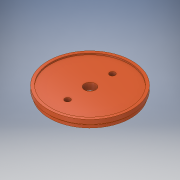
# Autodesk Inventor part: upper_thermal_barrier
Saved by Autodesk Inventor 2017 SP1 (Build 210196100, 196)
## iProperties
Created: 2016-10-21
Part Number: upper_thermal_barrier
Material: Phenolic Resin
Document SubType Name: Modeling
Designer: cflannery
Density: 1.38 g/cm^3
Appearance: Smooth - Light Orange
Author: cflannery
Autodesk Inventor part; units mm, degrees
ref_plane "YZ Plane" through (0, 0, 0) normal (1, 0, 0) x (0, 1, 0)
ref_plane "XZ Plane" through (0, 0, 0) normal (0, 1, 0) x (-1, 0, 0)
ref_plane "XY Plane" through (0, 0, 0) normal (0, 0, 1) x (1, 0, 0)
sketch "Sketch1" plane through (0, 0, 0) normal (0, 1, 0) x (-1, 0, 0)
  circle A0 centre (0, 0) radius 92.075
  dimension "d0" = 184.15
  constraints: 1 centre point, 1 coincident
  measures "d0" diameter of A0
extrude "Extrusion1" add sketch "Sketch1" along normal blind 6.35
sketch "Sketch2" plane through (0, 6.35, 0) normal (0, 1, 0) x (1, 0, 0)
  circle A0 centre (0, 0) radius 88.9
  dimension "d3" = 177.8
  constraints: 1 centre point, 1 coincident
  measures "d3" diameter of A0
extrude "Extrusion2" add sketch "Sketch2" along normal blind 3.175
sketch "Sketch3" plane through (0, 9.525, 0) normal (0, 1, 0) x (1, 0, 0)
  circle A0 centre (0, 0) radius 95.25
  dimension "d6" = 190.5
  constraints: 1 centre point, 1 coincident
  measures "d6" diameter of A0
extrude "Extrusion3" add sketch "Sketch3" along normal blind 6.35
sketch "Sketch8" plane through (0, 15.875, 0) normal (0, 1, 0) x (1, 0, 0)
  circle A0 centre (0, 0) radius 95.25
  circle A1 centre (0, 0) radius 88.9
  dimension "d33" = 177.8
  dimension "d34" = 190.5
  constraints: 2 centre point, 2 coincident
  measures "d33" diameter of A1
  measures "d34" diameter of A0
extrude "Extrusion9" add sketch "Sketch8" along normal blind 3.175
sketch "Sketch9" plane through (0, 15.875, 0) normal (0, 1, 0) x (1, 0, 0)
  circle A0 centre (0, 0) radius 12.7
  circle A1 centre (0, -50.8) radius 6.35
  circle A2 centre (0, 50.8) radius 6.35
  dimension "d37" = 12.7
  dimension "d38" = 50.8
  dimension "d39" = 50.8
  dimension "d40" = 25.4
  constraints: 3 centre point, 2 vertical alignment, 1 coincident, 1 equal radius
  measures "d37" diameter of A2
  measures "d38" distance of point (0, 0) A2.centre
  measures "d39" distance of A1.centre point (0, 0)
  measures "d40" diameter of A0
extrude "Extrusion10" cut sketch "Sketch9" against normal through all
body "Solid1"
